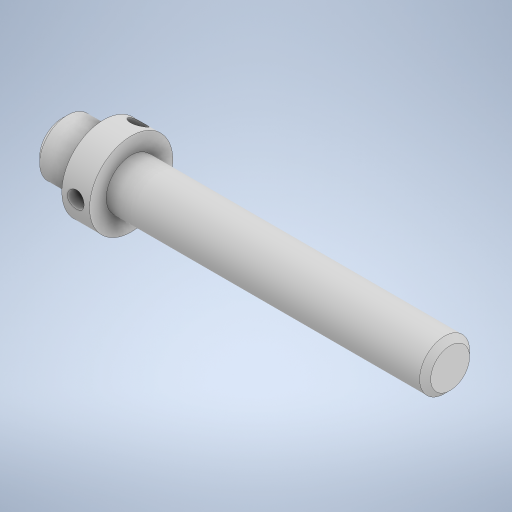
# Autodesk Inventor part: Coluna do Ferramental
Saved by Autodesk Inventor 2023 (Build 270158000, 158)
## iProperties
Created: 2022-04-25
Part Number: Coluna do Ferramental
Material: Generic
Document SubType Name: Modeling
Designer: coqui
Density: 1 g/cm^3
Appearance: Default
Author: coqui
Autodesk Inventor part; units mm, degrees
ref_plane "YZ Plane" through (0, 0, 0) normal (1, 0, 0) x (0, 1, 0)
ref_plane "XZ Plane" through (0, 0, 0) normal (0, 1, 0) x (-1, 0, 0)
sketch "Sketch1" plane through (0, 0, 0) normal (0, 0, 1) x (1, 0, 0)
  line L0 (0, 0) -> (-140, 0)
  line L1 (0, 0) -> (0, 7)
  line L2 (-2, 9) -> (-115, 9)
  line L3 (-115, 9) -> (-115, 15)
  line L4 (-115, 15) -> (-125, 15)
  line L5 (-125, 15) -> (-125, 10)
  line L6 (-125, 10) -> (-138, 10)
  line L7 (-140, 8) -> (-140, 0)
  line L8 (-138, 10) -> (-140, 8)
  line L9 (-2, 9) -> (0, 7)
  line L10 (-267.7899, 0) -> (-197.3543, 0) construction
  point P0 (0, 9)
  point P1 (-140, 10)
  point P2 (-120, 15)
  dimension "d1" = 140
  dimension "d2" = 15
  dimension "d3" = 10
  dimension "d4" = 15
  dimension "d5" = 9
  dimension "d6" = 10
  dimension "d7" = 2
  dimension "d8" = 2
  dimension "d9" = 2
  dimension "d10" = 2
  constraints: 22 end point, 5 perpendicular, 4 point on line, 3 horizontal, 1 midpoint, 1 vertical
  measures "d1" distance of L0.start L0.end
  measures "d2" distance of L5.end point (-140, 10)
  measures "d3" distance of L3.end L4.end
  measures "d4" vertical distance of L0.start point (-120, 15)
  measures "d5" distance of L0.start point (0, 9)
  measures "d6" distance of point (-140, 10) L0.end
  measures "d7" distance of L6.end point (-140, 10)
  measures "d8" distance of L7.start point (-140, 10)
  measures "d9" distance of L2.start point (0, 9)
  measures "d10" distance of L1.end point (0, 9)
revolve "Revolution1" add sketch "Sketch1" angle 360 about axis through (-267.7899, 0, 0) along (1, 0, 0)
ref_plane "Work Plane1" through (0, 0, 15) normal (0, 0, 1) x (1, 0, 0)
sketch "Sketch2" plane through (0, 0, 15) normal (0, 0, 1) x (1, 0, 0)
  circle A0 centre (-120, 0) radius 3
  line L0 (-115, -15) -> (-115, 15) projected
  point P0 (0, 0)
  dimension "d13" = 6
  dimension "d14" = 5
  constraints: 1 centre point
  measures "d13" diameter of A0
  measures "d14" distance from line of L0 A0.centre
extrude "Extrusion1" cut sketch "Sketch2" against normal blind 5
pattern_circular "Circular Pattern1" count 3 over 360 about axis through (-58.5, 0, 0) along (1, 0, 0) of "Extrusion1"
equation "\"d8\" = d7"
equation "\"d10\" = d9"
body "Solid1"
